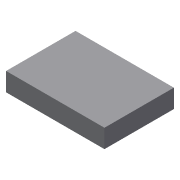
# Autodesk Inventor part: Battery
Saved by Autodesk Inventor 2020 (Build 240168000, 168)
## iProperties
Created: 2022-10-11
Part Number: Battery
Material: Allgemein
Document SubType Name: Modeling
Designer: uch10113
Density: 1 g/cm^3
Appearance: Vorgabe
Author: uch10113
Autodesk Inventor part; units mm, degrees
ref_plane "YZ Plane" through (0, 0, 0) normal (1, 0, 0) x (0, 1, 0)
ref_plane "XZ Plane" through (0, 0, 0) normal (0, 1, 0) x (-1, 0, 0)
ref_plane "XY Plane" through (0, 0, 0) normal (0, 0, 1) x (1, 0, 0)
sketch "Skizze1" plane through (0, 0, 0) normal (0, 0, 1) x (1, 0, 0)
  line L0 (-24.1948, 11.5325) -> (6.8052, 11.5325)
  line L1 (6.8052, 11.5325) -> (6.8052, -21.4675)
  line L2 (6.8052, -21.4675) -> (-24.1948, -21.4675)
  line L3 (-24.1948, -21.4675) -> (-24.1948, 11.5325)
  point P0 (0, 0)
  dimension "d0" = 33
  dimension "d1" = 31
  constraints: 8 end point, 2 parallel, 1 horizontal, 1 perpendicular
  measures "d0" distance of L2.end L0.start
  measures "d1" distance of L0.start L0.end
extrude "Extrusion1" add sketch "Skizze1" along normal blind 4
